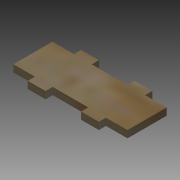
# Autodesk Inventor part: front(magi)
Saved by Autodesk Inventor 2015 (Build 190159000, 159)
## iProperties
Created: 2015-10-07
Part Number: front(magi)
Material: Generic
Document SubType Name: Modeling
Designer: Haukur
Density: 1 g/cm^3
Appearance: Plywood - Weathered
Author: Haukur
Autodesk Inventor part; units mm, degrees
ref_plane "YZ Plane" through (0, 0, 0) normal (1, 0, 0) x (0, 1, 0)
ref_plane "XZ Plane" through (0, 0, 0) normal (0, 1, 0) x (-1, 0, 0)
ref_plane "XY Plane" through (0, 0, 0) normal (0, 0, 1) x (1, 0, 0)
sketch "Sketch1" plane through (0, 0, 0) normal (0, 0, 1) x (1, 0, 0)
  line L0 (0, 4) -> (0, 26)
  line L1 (0, 26) -> (12.101, 26)
  line L2 (12.101, 26) -> (12.101, 30)
  line L3 (12.101, 30) -> (22.101, 30)
  line L4 (22.101, 30) -> (22.101, 26)
  line L5 (22.101, 26) -> (42.101, 26)
  line L6 (42.101, 26) -> (42.101, 30)
  line L7 (42.101, 30) -> (52.101, 30)
  line L8 (52.101, 30) -> (52.101, 26)
  line L9 (52.101, 26) -> (64.202, 26)
  line L10 (64.202, 26) -> (64.202, 4)
  line L11 (64.202, 4) -> (52.101, 4)
  line L12 (52.101, 4) -> (52.101, 0)
  line L13 (52.101, 0) -> (42.101, 0)
  line L14 (42.101, 0) -> (42.101, 4)
  line L15 (42.101, 4) -> (22.101, 4)
  line L16 (22.101, 4) -> (22.101, 0)
  line L17 (22.101, 0) -> (12.101, 0)
  line L18 (12.101, 0) -> (12.101, 4)
  line L19 (12.101, 4) -> (0, 4)
  point P0 (0, 0)
  dimension "d0" = 22
  dimension "d1" = 12.101
  dimension "d2" = 4
  dimension "d3" = 10
  dimension "d4" = 20
  dimension "d5" = 10
  dimension "d6" = 12.101
  constraints: 40 end point, 13 perpendicular, 12 point on line, 1 horizontal, 1 vertical
  measures "d0" distance of L0.start L0.end
  measures "d1" distance of L0.end L1.end
  measures "d2" distance of L1.end L2.end
  measures "d3" distance of L2.end L3.end
  measures "d4" distance of L4.end L5.end
  measures "d5" distance of L6.end L7.end
  measures "d6" distance of L8.end L9.end
extrude "Extrusion1" add sketch "Sketch1" along normal blind 4
body "Solid1"
